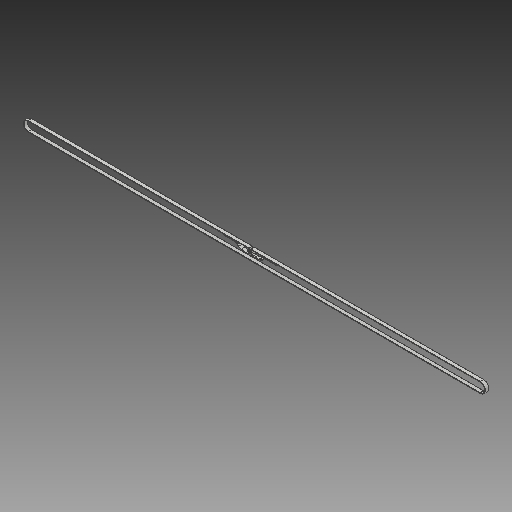
# Autodesk Inventor part: YBELT
Saved by Autodesk Inventor 2018 (Build 220112000, 112)
## iProperties
Created: 2016-07-22
Part Number: YBELT
Material: Generic
Document SubType Name: Modeling
Designer: User
Density: 1 g/cm^3
Appearance: Default
Author: User
Autodesk Inventor part; units mm, degrees
ref_plane "YZ Plane" through (0, 0, 0) normal (1, 0, 0) x (0, 1, 0)
ref_plane "XZ Plane" through (0, 0, 0) normal (0, 1, 0) x (-1, 0, 0)
ref_plane "XY Plane" through (0, 0, 0) normal (0, 0, 1) x (1, 0, 0)
sketch "Sketch1" plane through (0, 0, 0) normal (0, 0, 1) x (1, 0, 0)
  arc A0 (-16.0194, 6.752) -> (-16.0208, -6.1468) centre (-16.0175, 0.3026) ccw
  arc A1 (649.005, -6.4829) -> (649.0007, 6.9464) centre (649.0026, 0.2317) ccw
  line L0 (649.005, -6.4829) -> (-16.0208, -6.1468)
  arc A2 (649.0045, -7.4829) -> (649.0008, 7.9464) centre (649.0026, 0.2317) ccw
  line L1 (649.0008, 7.9464) -> (311.9827, 7.8478)
  line L2 (649.0045, -7.4829) -> (-16.0213, -7.1468)
  arc A3 (-16.0124, 7.7519) -> (-16.0213, -7.1468) centre (-16.0175, 0.3026) ccw
  line L3 (312.9758, 5.1048) -> (312.9758, 3.1737)
  line L4 (312.9758, 3.1737) -> (313.0166, 2.6809)
  line L5 (313.0166, 2.6809) -> (313.1377, 2.2016)
  line L6 (313.1377, 2.2016) -> (313.3359, 1.7486)
  line L7 (313.3359, 1.7486) -> (313.6059, 1.3343)
  line L8 (313.6059, 1.3343) -> (313.9402, 0.97)
  line L9 (313.9402, 0.97) -> (314.3298, 0.6656)
  line L10 (314.3298, 0.6656) -> (314.7641, 0.4293)
  line L11 (314.7641, 0.4293) -> (315.2314, 0.2675)
  line L12 (315.2314, 0.2675) -> (315.7189, 0.1847)
  line L13 (315.7189, 0.1847) -> (316.2133, 0.1831)
  line L14 (316.2133, 0.1831) -> (318.2319, 0.3939)
  line L15 (318.2319, 0.3939) -> (320.8327, 0.8165)
  line L16 (320.8327, 0.8165) -> (323.4008, 1.4058)
  line L17 (323.4008, 1.4058) -> (325.9257, 2.1591)
  line L18 (325.9257, 2.1591) -> (326.3565, 2.3413)
  line L19 (326.3565, 2.3413) -> (326.7537, 2.5883)
  line L20 (326.7537, 2.5883) -> (327.1077, 2.8941)
  line L21 (327.1077, 2.8941) -> (327.4099, 3.2511)
  line L22 (327.4099, 3.2511) -> (327.6529, 3.6508)
  line L23 (327.6529, 3.6508) -> (327.8308, 4.0834)
  line L24 (327.8308, 4.0834) -> (327.9394, 4.5384)
  line L25 (327.9394, 4.5384) -> (327.9758, 5.0047)
  line L26 (327.9758, 5.1048) -> (327.9758, 5.0047)
  line L27 (312.9758, 5.1048) -> (327.9758, 5.1048)
  line L28 (308.2722, 6.8467) -> (308.2722, 3.2511)
  line L29 (308.2722, 3.2511) -> (307.9758, 1.1103)
  line L30 (307.9758, 1.1103) -> (306.659, 0.0522)
  line L31 (306.659, 0.0522) -> (304.4805, -0.3835)
  line L32 (304.4805, -0.3835) -> (297.6339, 0.7991)
  line L33 (297.6339, 0.7991) -> (293.4637, 2.2307)
  line L34 (293.4637, 2.2307) -> (291.5964, 4.3469)
  line L35 (291.5964, 4.3469) -> (289.9159, 5.7785)
  line L36 (289.9159, 5.7785) -> (288.4843, 6.3387)
  line L37 (288.4843, 6.3387) -> (285.1855, 6.4631)
  line L38 (285.1855, 6.4631) -> (276.9073, 6.3387)
  line L39 (276.9073, 6.3387) -> (272.4922, 5.7434)
  line L40 (272.4922, 5.7434) -> (272.7903, 5.0479)
  line L41 (272.7903, 5.0479) -> (277.3612, 5.5944)
  line L42 (277.3612, 5.5944) -> (285.9563, 5.7931)
  line L43 (285.9563, 5.7931) -> (288.9373, 5.5944)
  line L44 (288.9373, 5.5944) -> (290.6266, 4.4517)
  line L45 (290.6266, 4.4517) -> (291.4215, 3.1599)
  line L46 (291.4215, 3.1599) -> (293.4088, 1.3216)
  line L47 (293.4088, 1.3216) -> (297.5325, 0.0795)
  line L48 (297.5325, 0.0795) -> (302.7492, -0.9638)
  line L49 (302.7492, -0.9638) -> (305.929, -1.0135)
  line L50 (305.929, -1.0135) -> (308.7609, 0.1789)
  line L51 (308.7609, 0.1789) -> (309.4068, 2.0172)
  line L52 (309.4068, 2.0172) -> (309.3584, 4.7043)
  line L53 (309.3584, 4.7043) -> (309.1601, 6.2436)
  line L54 (309.1601, 6.2436) -> (308.9658, 7.7519)
  line L55 (312.672, 6.848) -> (312.672, 3.2511)
  line L56 (312.672, 3.2511) -> (312.9684, 1.1103)
  line L57 (312.9684, 1.1103) -> (314.2852, 0.0522)
  line L58 (314.2852, 0.0522) -> (316.4637, -0.3835)
  line L59 (316.4637, -0.3835) -> (323.3103, 0.7991)
  line L60 (323.3103, 0.7991) -> (327.4805, 2.2307)
  line L61 (327.4805, 2.2307) -> (329.3478, 4.3469)
  line L62 (329.3478, 4.3469) -> (331.0283, 5.7785)
  line L63 (331.0283, 5.7785) -> (332.4599, 6.3387)
  line L64 (332.4599, 6.3387) -> (335.7587, 6.4631)
  line L65 (335.7587, 6.4631) -> (344.0369, 6.3387)
  line L66 (344.0369, 6.3387) -> (348.452, 5.7434)
  line L67 (348.452, 5.7434) -> (348.156, 5.0487)
  line L68 (348.156, 5.0487) -> (343.5851, 5.5953)
  line L69 (343.5851, 5.5953) -> (334.9899, 5.794)
  line L70 (334.9899, 5.794) -> (332.009, 5.5953)
  line L71 (332.009, 5.5953) -> (330.3197, 4.4525)
  line L72 (330.3197, 4.4525) -> (329.5248, 3.1608)
  line L73 (329.5248, 3.1608) -> (327.5375, 1.3225)
  line L74 (327.5375, 1.3225) -> (323.4138, 0.0804)
  line L75 (323.4138, 0.0804) -> (318.197, -0.9629)
  line L76 (318.197, -0.9629) -> (315.0173, -1.0126)
  line L77 (315.0173, -1.0126) -> (312.1854, 0.1798)
  line L78 (312.1854, 0.1798) -> (311.5395, 2.0181)
  line L79 (311.5395, 2.0181) -> (311.5892, 4.8003)
  line L80 (311.5892, 4.8003) -> (311.7879, 6.3395)
  line L81 (311.5892, 4.8003) -> (311.9827, 7.8478)
  line L82 (-16.0194, 6.752) -> (308.2722, 6.8467)
  line L83 (312.672, 6.848) -> (649.0007, 6.9464)
  line L84 (308.9658, 7.7519) -> (-16.0124, 7.7519)
  point P0 (0, 0)
  dimension "d1" = 1
  constraints: 170 end point, 9 point on circle, 4 centre point, 4 point on line
  measures "d1" distance between parallel lines of L0 L2
extrude "Extrusion1" add sketch "Sketch1" along normal blind 5 contours A0 L0 A1 L83 L55 L56 L57 L58 L59 L60 L61 L62 L63 L64 L65 L66 L67 L68 L69 L70 L71 L72 L73 L74 L75 L76 L77 L78 L79 L80 L81 L1 A2 L2 A3 L84 L54 L53 L52 L51 L50 L49 L48 L47 L46 L45 L44 L43 L42 L41 L40 L39 L38 L37 L36 L35 L34 L33 L32 L31 L30 L29 L28 L82
body "Solid1"
